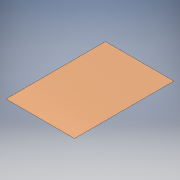
# Autodesk Inventor part: Floor
Saved by Autodesk Inventor 2016 (Build 200138000, 138)
## iProperties
Created: 2016-01-13
Part Number: Floor
Material: Wood (Birch)
Document SubType Name: Modeling
Designer: Douglas
Density: 0.55 g/cm^3
Appearance: Birch - Natural Polished
Author: Douglas
Autodesk Inventor part; units mm, degrees
ref_plane "YZ Plane" through (0, 0, 0) normal (1, 0, 0) x (0, 1, 0)
ref_plane "XZ Plane" through (0, 0, 0) normal (0, 1, 0) x (-1, 0, 0)
ref_plane "XY Plane" through (0, 0, 0) normal (0, 0, 1) x (1, 0, 0)
sketch "Sketch1" plane through (0, 0, 0) normal (0, 1, 0) x (-1, 0, 0)
  line L0 (0, 0) -> (42461.4778, 0)
  line L1 (42461.4778, 0) -> (42461.4778, -61660.2297)
  line L2 (42461.4778, -61660.2297) -> (0, -61660.2297)
  line L3 (0, -61660.2297) -> (0, 0)
  constraints: 8 end point, 2 parallel, 1 horizontal, 1 perpendicular
extrude "Extrusion1" add sketch "Sketch1" along normal blind 3.175
body "Solid1"
